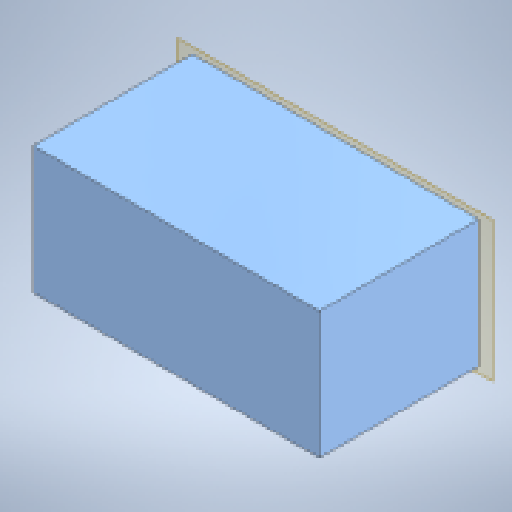
# Autodesk Inventor part: Acuario
Saved by Autodesk Inventor 2024 (Build 280153000, 153)
## iProperties
Created: 2024-04-05
Part Number: Acuario
Material: Genérico
Document SubType Name: Modeling
Designer: sergi
Density: 1 g/cm^3
Appearance: Valor por defecto
Author: sergi
Autodesk Inventor part; units mm, degrees
ref_plane "YZ Plane" through (0, 0, 0) normal (1, 0, 0) x (0, 1, 0)
ref_plane "XZ Plane" through (0, 0, 0) normal (0, 1, 0) x (-1, 0, 0)
ref_plane "XY Plane" through (0, 0, 0) normal (0, 0, 1) x (1, 0, 0)
ref_plane "Plano de trabajo1" through (0, 0, 0) normal (0, 0, 1) x (1, 0, 0)
sketch "Boceto1" plane through (0, 0, 0) normal (0, 0, 1) x (1, 0, 0)
  line L0 (450, 200) -> (-450, 200) projected
  line L1 (-450, 200) -> (-450, -200) projected
  line L2 (-450, -200) -> (450, -200) projected
  line L3 (450, -200) -> (450, 200) projected
  point P0 (0, 0)
extrude "Extrusión1" add sketch "Boceto1" along normal blind 500
